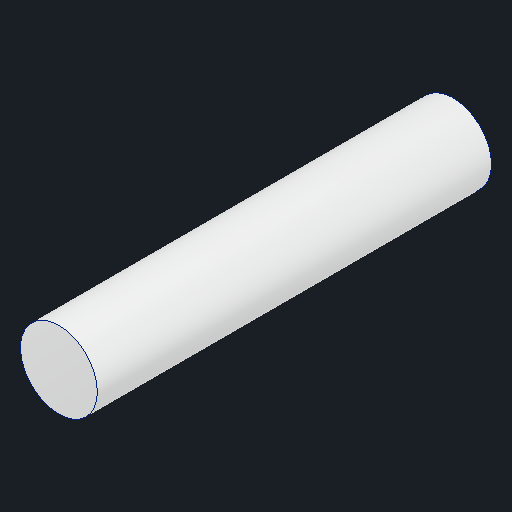
# Autodesk Inventor part: smolGear_shaft
Saved by Autodesk Inventor 2023 (Build 270158000, 158)
## iProperties
Created: 2024-04-14
Part Number: smolGear_shaft
Material: Aluminum 6061
Document SubType Name: Modeling
Designer: szymo
Density: 27.8521 g/cm^3
Appearance: Aluminum - Flat
Mass: 7 g
Surface Area: 2.7646 cm^2
Volume: 0.251327 cm^3
TOTAL MASS: 0.0
Author: szymo
Autodesk Inventor part; units mm, degrees
note: some values were not read from the file. Chosen so that the rebuilt part matches the saved one: second side of "Extrusion1".
ref_plane "Work Plane1" through (0, 0, 0) normal (0, 0, 1) x (1, 0, 0)
sketch "Sketch1" plane through (0, 0, 0) normal (0, 0, 1) x (1, 0, 0)
  circle A0 centre (54.3953, -16.1803) radius 4.0005 projected
  circle A1 centre (54.3953, -16.1803) radius 2
  point P0 (0, 0)
  constraints: 1 centre point, 2 other
ref_plane "Work Plane2" through (0, -29.5, -27) normal (0, 0, -1) x (0, 1, 0)
ref_plane "Work Plane3" through (38.9126, -31.7019, -38) normal (0, 0, -1) x (0.3642575, 0.9312983, 0)
extrude "Extrusion1" add sketch "Sketch1" along normal blind 20.5 contours A1
body "Solid1"
